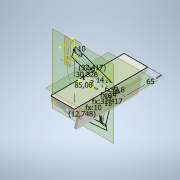
# Autodesk Inventor part: Capping_RotationAnchor
Saved by Autodesk Inventor 2022 (Build 260153000, 153)
## iProperties
Created: 2024-05-05
Part Number: Capping_RotationAnchor
Material: Generic
Document SubType Name: Modeling
Designer: raphael.hauk
Density: 1 g/cm^3
Appearance: Default
Author: raphael.hauk
Autodesk Inventor part; units mm, degrees
ref_plane "YZ Plane" through (0, 0, 0) normal (1, 0, 0) x (0, 1, 0)
ref_plane "XZ Plane" through (0, 0, 0) normal (0, 1, 0) x (-1, 0, 0)
ref_plane "XY Plane" through (0, 0, 0) normal (0, 0, 1) x (1, 0, 0)
ref_plane "Work Plane6" through (7.98, 0, 4.3086) normal (0, 0, 1) x (1, 0, 0)
sketch "Sketch1" plane through (0, 0, 0) normal (0, 0, 1) x (1, 0, 0)
  line L0 (7.98, 8) -> (7.98, -8) projected
  line L1 (7.98, 8) -> (3.98, 8) projected
  line L2 (3.98, -8) -> (3.98, 8) projected
  line L3 (7.98, -8) -> (3.98, -8) projected
  point P0 (0, 0)
  point P1 (21.25, -8.826)
  constraints: 2 other
sketch "Sketch2" plane through (0, 0, 0) normal (0, 0, 1) x (1, 0, 0)
  line L0 (20.7277, -44.9331) -> (36.6668, -43.5386)
  line L1 (36.6668, -43.5386) -> (37.0155, -47.5234)
  line L2 (37.0155, -47.5234) -> (21.0763, -48.9179)
  line L3 (21.0763, -48.9179) -> (20.7277, -44.9331)
  line L4 (3.98, -8) -> (3.98, 8) construction
  line L5 (7.98, 8) -> (3.98, 8) construction
  line L6 (7.98, 8) -> (7.98, -8) construction
  line L7 (7.98, -8) -> (3.98, -8) construction
  line L8 (38.606, -12.626) -> (7.98, -2) construction
  line L9 (30.6897, -44.0616) -> (38.606, -12.626) construction
  arc A0 (7.98, 8) -> (20.7277, -44.9331) centre (38.606, -12.626) ccw construction
  line L10 (21.25, -8.826) -> (0, -8.826) construction
  line L11 (8.9996, 2.9386) -> (40.245, -7.9022)
  line L12 (40.245, -7.9022) -> (36.967, -17.3498)
  line L13 (36.967, -17.3498) -> (5.7217, -6.5089)
  line L14 (5.7217, -6.5089) -> (8.9996, 2.9386)
  line L15 (8.9996, 2.9386) -> (36.967, -17.3498) construction
  line L16 (40.245, -7.9022) -> (5.7217, -6.5089) construction
  line L17 (38.606, -12.626) -> (30.6897, -44.0616)
  line L18 (30.6897, -44.0616) -> (35.5383, -45.2826)
  line L19 (35.5383, -45.2826) -> (43.4546, -13.847)
  line L20 (43.4546, -13.847) -> (38.606, -12.626)
  point P0 (35.1872, -26.2021)
  point P1 (25.3795, -8.0369)
  point P2 (22.9833, -7.2056)
  point P3 (7.98, 0)
  dimension "d3" = 10
  dimension "d5" = 10
  dimension "d6" = 32.417
  dimension "d7" = 32.417
  dimension "d8" = 3.8
  dimension "d9" = 30.626
  dimension "d26" = 14
  dimension "d27" = 14
  dimension "d44" = 10
  dimension "d47" = 5
  dimension "d82" = 12.7477
  dimension "d83" = 85
  constraints: 34 end point, 7 parallel, 6 point on line, 4 midpoint, 3 perpendicular, 2 equal length, 2 point on circle, 1 centre point, 1 coincident, 1 collinear, 1 horizontal
  measures "d3" distance of L5.start L8.end
  measures "d5" distance of L0.start L9.start
  measures "d6" distance of L8.start L8.end
  measures "d7" distance of L9.start L8.start
  measures "d8" distance from line of L17.start L10
  measures "d9" distance from line of L6 L17.start
  measures "d26" distance of point (25.379, -8.037) L17.start
  measures "d27" distance of point (35.187, -26.202) L17.start
  measures "d44" distance of L11.end L12.end
  measures "d47" distance of L19.end L17.start
  measures "d82" horizontal distance of L0.start L6.end
  measures "d83" angle of L0 L6
ref_plane "Work Plane1" through (18.228, -8.826, 23.9001) normal (0, -1, 0) x (0, 0, -1)
sketch "Sketch3" plane through (18.228, -8.826, 23.9001) normal (0, -1, 0) x (0, 0, -1)
  circle A0 centre (11.5, 16.822) radius 1.45 construction
  circle A1 centre (26.5, 16.822) radius 1.45 construction
  circle A2 centre (11.5, 6.822) radius 1.45 construction
  circle A3 centre (26.5, 6.822) radius 1.45 construction
  line L0 (-12.9085, 5.822) -> (52.0915, 5.822)
  line L1 (52.0915, 5.822) -> (52.0915, 26.822)
  line L2 (52.0915, 26.822) -> (-12.9085, 26.822)
  line L3 (-12.9085, 26.822) -> (-12.9085, 5.822)
  line L4 (19.5915, -18.302) -> (19.5915, 38.076) construction
  point P0 (23.9001, -18.228)
  dimension "d10" = 10
  dimension "d11" = 1
  dimension "d55" = 65
  constraints: 10 end point, 2 parallel, 1 horizontal, 1 perpendicular, 1 vertical, 3 other
  measures "d10" distance from line of L2 A0.centre
  measures "d11" distance from line of L0 A2.centre
  measures "d55" distance of L1.end L2.end
extrude "Extrusion1" add sketch "Sketch3" along normal blind 2
ref_plane "Work Plane3" through (18.228, -12.826, 23.9001) normal (0, -1, 0) x (1, 0, 0)
sketch "Sketch4" plane through (18.228, -12.826, 23.9001) normal (0, -1, 0) x (1, 0, 0)
  point P0 (-18.228, -23.9001)
  point P1 (6.822, -11.5)
  point P2 (6.822, -26.5)
  point P3 (16.822, -11.5)
  point P4 (16.822, -26.5)
sketch "Sketch5" plane through (29.03, -8.826, 4.3086) normal (0, 0, 1) x (1, 0, 0)
  circle A0 centre (9.576, -3.8) radius 1.5
  line L0 (-4.98, -2) -> (16.02, -2) projected
  arc A1 (8.5926, -6.6343) -> (12.4852, -4.5326) centre (9.576, -3.8) ccw
  line L1 (7.937, -8.5238) -> (-23.3083, 2.3171) construction
  line L2 (7.937, -8.5238) -> (-6.2342, -3.6069) construction
  line L3 (-6.2342, -3.6069) -> (-5.5786, -1.7174) construction
  line L4 (-5.5786, -1.7174) -> (8.5926, -6.6343) construction
  line L5 (8.5926, -6.6343) -> (7.937, -8.5238) construction
  line L6 (-5.5786, -1.7174) -> (8.5926, -6.6343)
  line L7 (6.5083, -36.4566) -> (14.4246, -5.021) construction
  line L8 (14.4246, -5.021) -> (10.7616, -19.5669) construction
  line L9 (10.7616, -19.5669) -> (8.8221, -19.0785) construction
  line L10 (8.8221, -19.0785) -> (12.4852, -4.5326) construction
  line L11 (12.4852, -4.5326) -> (14.4246, -5.021)
  arc A2 (8.5926, -6.6343) -> (12.4852, -4.5326) centre (9.576, -3.8) ccw construction
  line L12 (14.4246, -5.021) -> (16.02, -2)
  line L13 (-4.98, -2) -> (-4.98, -1.9251)
  point P0 (-29.03, 8.826)
  point P1 (9.576, -3.8)
  point P2 (12.4103, -4.7834)
  point P3 (-4.7641, -2)
  dimension "d21" = 3
  dimension "d46" = 2
  dimension "d70" = 15
  constraints: 22 end point, 7 equal length, 5 point on line, 4 point on circle, 3 centre point, 3 coincident, 2 perpendicular, 1 tangent, 1 vertical
  measures "d21" diameter of A0
  measures "d46" distance between parallel lines of L1 L4
  measures "d70" distance of L9.end L10.end
extrude "Extrusion2" add sketch "Sketch5" along normal mid plane 65 contours A0 | L0 L12 L11 A1 L6
ref_plane "Work Plane5" through (45.05, -8.826, 4.3086) normal (0, 0, -1) x (-1, 0, 0)
sketch "Sketch7" plane through (45.05, -8.826, 4.3086) normal (0, 0, -1) x (-1, 0, 0)
  line L0 (0, -2) -> (3.319, -20.0553)
  line L1 (3.319, -20.0553) -> (5.2584, -19.5669)
  line L2 (1.5954, -5.021) -> (5.2584, -19.5669) construction
  line L3 (0, 0) -> (0, -2) construction
  line L4 (0, -2) -> (1.5954, -5.021)
  line L5 (5.2584, -19.5669) -> (1.5954, -5.021)
  line L6 (0, -2) -> (1.5954, -5.021) projected
  line L7 (0, -2) -> (0, -6.8757)
  line L8 (0, -6.8757) -> (3.319, -20.0553)
  point P0 (45.05, 8.826)
  point P1 (0, -2)
  dimension "d66" = 2
  constraints: 12 end point, 1 coincident, 1 collinear, 1 parallel, 1 perpendicular, 1 vertical
  measures "d66" distance between parallel lines of L8 L2
extrude "Extrusion3" add sketch "Sketch7" along normal mid plane 55
hole "Hole1" at (35.05, -12.826, 12.4001) at (35.05, -12.826, -2.5999) direction (0, 1, 0) diameter 2.6 end through all start extended yes counterbore diameter 5.5 counterbore depth 2 clearance for "Socket Head Cap Screw ISO 4762" size "M2.5" standard "ISO"
fillet "Fillet1" radius 1 2 edges at (44.2523, -12.3365, 31.8086) (44.2523, -12.3365, -23.1914)
sketch "Sketch8" plane through (37.6226, -15.4603, -28.1914) normal (-0.3277907, -0.9447504, 0) x (0.9447504, -0.3277907, 0)
  circle A0 centre (-8, 50.5) radius 5
  line L0 (30.9204, 32.5) -> (-59.6333, 32.5) projected
  line L1 (0, 26.5631) -> (0, 39.6199) projected
  point P0 (-40.6117, 28.1914)
  dimension "d56" = 10
  dimension "d57" = 8
  dimension "d84" = 18
  constraints: 1 centre point
  measures "d56" diameter of A0
  measures "d57" distance from line of A0.centre L1
  measures "d84" distance from line of L0 A0.centre
extrude "Extrusion4" cut sketch "Sketch8" against normal blind 1.2
sketch "Sketch9" plane through (39.7916, -28.3929, -23.1914) normal (-0.9697242, 0.2442029, 0) x (0, 0, 1)
  circle A0 centre (45.5, 7) radius 4.925
  line L0 (27.5, -43.9342) -> (27.5, 49.9934) projected
  line L1 (-5, 15) -> (-1, 15) projected
  line L2 (-1, 15) -> (56, 15) projected
  point P0 (23.1914, 17.816)
  point P1 (27.5, 15)
  point P2 (0, 15)
  dimension "d60" = 9.85
  dimension "d85" = 18
  dimension "d87" = 8
  constraints: 1 centre point
  measures "d60" diameter of A0
  measures "d85" distance from line of L0 A0.centre
  measures "d87" distance from line of A0.centre L2
extrude "Extrusion5" cut sketch "Sketch9" against normal blind 1.2
draft "FaceDraft1" angle 5 pull direction (0.9697242, -0.2442029, 0) faces at (42.1813, -22.1848, 27.2177) fixed edges at (41.501, -21.6048, 17.3836)
draft "FaceDraft2" angle 5 pull direction (0.3277907, 0.9447504, 0) faces at (34.8585, -14.0771, 21.5066) fixed edges at (25.3409, -11.199, 22.3086)
mirror "Mirror2" about plane through (45.05, -8.826, 4.3086) normal (0, 0, -1) of "Extrusion5", "Extrusion4", "FaceDraft1", "FaceDraft2"
sketch "Sketch10" plane through (24.05, -8.826, 36.8086) normal (0, 0, 1) x (1, 0, 0)
  point P0 (-24.05, 8.826)
  point P1 (14.556, -3.8)
hole "Hole2" at (38.606, -12.626, 36.8086) direction (0, 0, -1) diameter 2.1 depth 12 tip angle 118 clearance for "Socket Head Cap Screw ISO 4762" size "M2" standard "ISO"
ref_plane "Work Plane7" through (24.05, -8.826, 34.8086) normal (0, 0, 1) x (1, 0, 0)
sketch "Sketch11" plane through (24.05, -8.826, 34.8086) normal (0, 0, 1) x (1, 0, 0)
  circle A0 centre (14.556, -3.8) radius 1.05 projected
  line L0 (12.531, -2.6309) -> (14.556, -1.4617)
  line L1 (14.556, -1.4617) -> (16.581, -2.6309)
  line L2 (16.581, -2.6309) -> (16.581, -4.9691)
  line L3 (16.581, -4.9691) -> (14.556, -6.1383) construction
  line L4 (14.556, -6.1383) -> (12.531, -4.9691) construction
  line L5 (12.531, -4.9691) -> (12.531, -2.6309)
  line L6 (16.581, -4.9691) -> (16.581, -6.0135)
  arc A1 (13.5726, -6.6343) -> (17.4652, -4.5326) centre (14.556, -3.8) ccw projected
  line L7 (12.531, -4.9691) -> (12.531, -6.2728)
  line L8 (0.2159, -2) -> (13.5726, -6.6343) projected
  point P0 (-24.05, 8.826)
  point P1 (20.3903, -4.7834)
  point P2 (0, -2.2721)
  dimension "d79" = 4.05
  constraints: 16 end point, 3 vertical, 1 coincident, 1 point on circle, 15 other
  measures "d79" distance between parallel lines of L5 L2
extrude "Extrusion6" cut sketch "Sketch11" against normal blind 1.63 contours A0 | L0 L1 L2 L6 A1 L8 L7 L5
mirror "Mirror1" about plane through (45.05, -8.826, 4.3086) normal (0, 0, -1) of "Extrusion6", "Hole2"
equation "\"d5\" = d3"
equation "\"d7\" = d6"
equation "\"d27\" = d26"
equation "\"d47\" = 0.5 * d44"
body "Solid1"
